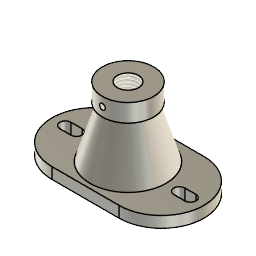
Swivel Bearing_ (Autodesk Fusion 360 archive; units mm, degrees)
design "Body"
Autodesk Fusion 360 part; units mm, degrees
sketch "Sketch1" plane through (0, 0, 0) normal (0, 0, 1) x (1, 0, 0)
  circle A0 centre (0, 0) radius 24
  line L0 (30, 38) -> (-30, 38)
  arc A1 (-30, 38) -> (-30, -38) centre (-30, 0) ccw
  line L1 (-30, -38) -> (30, -38)
  arc A2 (30, -38) -> (30, 38) centre (30, 0) ccw
  line L2 (30, 0) -> (-30, 0) construction
  dimension "d1" = 48
  dimension "d2" = 60
  dimension "d3" = 38
  constraint coincident A0.centre origin
  constraint tangent L0 A1
  constraint tangent A1 L1
  constraint parallel L0 L1
  constraint tangent L1 A2
  constraint tangent L0 A2
  constraint horizontal L2
  constraint midpoint L2 A0.centre
  measures "d1" diameter of A0
  measures "d2" distance of A2.centre A1.centre
  measures "d3" radius of A1
extrude "Extrude1" add sketch "Sketch1" along normal blind 10 makes body 1
sketch "Sketch2" plane through (0, 0, 0) normal (0, 1, 0) x (1, 0, 0)
  line L0 (0, 0) -> (0, -78.5429) construction
  line L1 (24, -10.0113) -> (11, -52.0077)
  line L2 (11, -52.0077) -> (11, -72.0077)
  line L3 (11, -72.0077) -> (23, -72.0077)
  line L4 (23, -72.0077) -> (23, -56.0077)
  line L5 (23, -56.0077) -> (21.8093, -56.0077)
  line L6 (20.3764, -54.0641) -> (34, -10.0531)
  line L7 (34, -10.0531) -> (24, -10.0113)
  arc A0 (20.3764, -54.0641) -> (21.8093, -56.0077) centre (21.8093, -54.5077) ccw
  dimension "d6" = 20
  dimension "d7" = 16
  dimension "d8" = 22
  dimension "d9" = 46
  dimension "d10" = 24
  dimension "d11" = 10
  dimension "d13" = 62
  dimension "d14" = 1.5
  constraint coincident L0.start origin
  constraint vertical L0
  constraint parallel L0 L2
  constraint perpendicular L2 L3
  constraint perpendicular L3 L4
  constraint perpendicular L4 L5
  constraint parallel L1 L6
  constraint tangent L5 A0
  constraint tangent L6 A0
  measures "d6" distance of L1.end L2.end
  measures "d7" distance of L3.end L4.end
  measures "d10" horizontal distance of L0.start L1.start
  measures "d11" horizontal distance of L1.start L6.end
  measures "d13" distance of L3.end L7
  measures "d14" radius of A0
revolve "Revolve1" add sketch "Sketch2" angle 360 about axis through (0, 0, 0) along (0, 0, 1) separate body makes body 2
sketch "Sketch3" plane through (0, 0, 10) normal (0, 0, 1) x (-1, 0, 0)
  circle A0 centre (0, 0) radius 24
  arc A1 (-30, 38) -> (-30, -38) centre (-30, 0) ccw
  line L0 (-30, -38) -> (30, -38)
  arc A2 (30, -38) -> (30, 38) centre (30, 0) ccw
  line L1 (30, 38) -> (-30, 38)
  line L2 (0, 0) -> (0, 62.4779) construction
  line L3 (-46, 5.0523) -> (-56, 5.0523)
  arc A3 (-56, 5.0523) -> (-56, -4.9477) centre (-56, 0.0523) ccw
  line L4 (-56, -4.9477) -> (-46, -4.9477)
  arc A4 (-46, -4.9477) -> (-46, 5.0523) centre (-46, 0.0523) ccw
  line L5 (-46, 0.0523) -> (-56, 0.0523) construction
  line L6 (56, -4.9477) -> (46, -4.9477)
  arc A5 (46, 5.0523) -> (46, -4.9477) centre (46, 0.0523) ccw
  line L7 (46, 5.0523) -> (56, 5.0523)
  arc A6 (56, -4.9477) -> (56, 5.0523) centre (56, 0.0523) ccw
  point P0 (-51, 0.0523)
  dimension "d16" = 51
  dimension "d17" = 10
  dimension "d18" = 5
  constraint coincident A0.centre L2.start
  constraint vertical L2
  constraint tangent L3 A3
  constraint tangent A3 L4
  constraint parallel L3 L4
  constraint tangent L4 A4
  constraint tangent L3 A4
  constraint horizontal L5
  constraint midpoint L5 P0
  constraint symmetric L2 L3.start A5.start
  constraint symmetric L2 L3.end L7.end
  constraint symmetric L2 A3.end L6.start
  constraint symmetric L2 L4.end L6.end
  constraint symmetric L2 A3 A6
  constraint symmetric L2 A4 A5
  measures "d16" horizontal distance of A0.centre P0
  measures "d17" distance of A3.end L4.end
  measures "d18" radius of A3
extrude "Extrude2" cut sketch "Sketch3" against normal blind 115 contours L3 A3 L4 A4 | L6 A5 L7 A6 bodies 1
sketch "Sketch4" plane through (0, 0, 0) normal (0, 1, 0) x (1, 0, 0)
  circle A0 centre (0, -64.0077) radius 3
  point P0 (23, -72.0077)
  dimension "d21" = 6
  dimension "d22" = 8
  measures "d21" diameter of A0
  measures "d22" vertical distance of A0.centre P0
extrude "Extrude3" cut sketch "Sketch4" against normal blind 35 bodies 2
thread "Thread1" "ISO Metric profile 22.0 M22x3 M22x3 6H" major diameter 22.3386 minor diameter 19.0024 pitch 3 angle 60 resizes the face on face at (10.9453, -1.0952, 65.341) on bodies 2
thread "Thread2" "ISO Metric profile 6.0 M6x1 M6x1 6H" major diameter 6.147 minor diameter 5.035 pitch 1 angle 60 resizes the face on face at (2.9871, -18.2116, 63.7295) on bodies 2

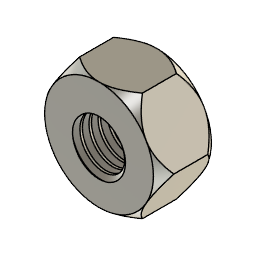
design "Nut"
Autodesk Fusion 360 part; units mm, degrees
sketch "Sketch1" plane through (0, 0, 0) normal (0, 1, 0) x (1, 0, 0)
  circle A0 centre (0, 0) radius 4
  line L0 (4.3301, -7.5) -> (8.6603, 0)
  line L1 (8.6603, 0) -> (4.3301, 7.5)
  line L2 (4.3301, 7.5) -> (-4.3301, 7.5)
  line L3 (-4.3301, 7.5) -> (-8.6603, 0)
  line L4 (-8.6603, 0) -> (-4.3301, -7.5)
  line L5 (-4.3301, -7.5) -> (4.3301, -7.5)
  dimension "d1" = 8
  dimension "d2" = 15
  constraint coincident A0.centre origin
  constraint horizontal L3.end A0.centre
  measures "d1" diameter of A0
  measures "d2" distance of L2 L5
extrude "Extrude1" add sketch "Sketch1" along normal mid plane 8
sketch "Sketch2" plane through (0, -4, 0) normal (0, -1, 0) x (1, 0, 0)
  circle A0 centre (0, 0) radius 4
  line L0 (4.3301, 7.5) -> (-4.3301, 7.5)
  line L1 (-4.3301, 7.5) -> (-8.6603, 0)
  line L2 (-8.6603, 0) -> (-4.3301, -7.5)
  line L3 (-4.3301, -7.5) -> (4.3301, -7.5)
  line L4 (4.3301, -7.5) -> (8.6603, 0)
  line L5 (8.6603, 0) -> (4.3301, 7.5)
  circle A1 centre (0, 0) radius 7.5
  dimension "d5" = 15
  constraint coincident A0.centre A1.centre
  measures "d5" diameter of A1
extrude "Extrude2" cut sketch "Sketch2" against normal through all of body 1 draft 35 contours A1 keep common part
mirror "Mirror1" about plane through (0, 0, 0) normal (0, 1, 0) of "Extrude2"
thread "Thread1" "ISO Metric profile 8.0 M8x1.25 M8x1.25 6H" major diameter 8.17 minor diameter 6.7795 pitch 1.25 angle 60 modelled right hand crest width 0.343 on face at (3.995, 1.3333, 0.1994) crest through (3.3898, -3.6875, 0)
